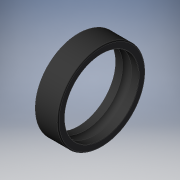
# Autodesk Inventor part: SKF_618/6_PART2
Saved by Autodesk Inventor 2019 (Build 230136000, 136)
## iProperties
Created: 2022-10-05
Part Number: SKF_618/6_PART2
Material: Generic
Catalog Web Link: www.cadenas.de
Description: -Deep groove ball bearings
Vendor: SKF
Document SubType Name: Modeling
Designer: psAdmin
Manufacturer: SKF
Mass: 4 g
Surface Area: 3.38269 cm^2
Volume: 0.123541 cm^3
Density: 1 g/cm^3
Appearance: PSOLRGB-175-175-175
Category: PARTsolutions
Company: SKF
Title: SKF_618/6_PART2
Author: Cadenas PARTsolutions
Comments: Deep groove ball bearings
PSOL_IDENT_0: {$CADENAS_DATA/23d-libs/skf/bearings_units_and_housings/ball_bearings/deep_groove_ball_bearings/bb1_
PSOL_IDENT_1: 001_101.prj},196 {VTYP=3D},{NB=SKF_618/6_PART2},{LINA=SKF_618/6_PART2},{NN=BB1_001_101_PART2},{NOPRJ=
PSOL_IDENT_2: TRUE},{DATE=09.09.2022 10:31:03},{GEOMDATE=07.09.2022 12:28:28},{VERSION=},{LINEID=8510},{WBVAR=},{W
PSOL_IDENT_3: BNUMERIC=}  {NB=SKF_618/6_PART2},{LINA=SKF_618/6_PART2},{KT=DUMMY},{DESIGNATION=618/6},{R12=0.15},{D
PSOL_IDENT_4: D=6.000},{D=13.000},{B=3.500},{C=},{CX=},{CXX=},{CA=0.000},{XXVARIANT=},{XXDESIGN=Single row},{XXSEA
PSOL_IDENT_5: LING=No seals},{DESIGN=dgbb1},{DESIGNIR=dgbb1},{VARIANT=},{DD1=8.00},{DD2=},{DD2X=},{DD2A=0.00},{D1=
PSOL_IDENT_6: 11.00},{D1X=0.00},{D2=},{D2A=0.00},{D3=},{D3X=},{D3A=0.000},{D4=},{HH=0.000},{BB=0.000},{BBX=},{BBA=
PSOL_IDENT_7: 0.000},{FF=},{R0MAX=0.000},{R0=0.000},{PITCH=9.50},{DW=2.000},{DDAMIN=6.800},{DDAMAX=0.000},{DDBMIN=
PSOL_IDENT_8: 0.000},{DDBMAX=0.000},{DBMIN=0.000},{DAMAX=12.200},{BBAMIN=0.000},{CAMAX=0.000},{RAMAX=0.100},{LOAD1=
PSOL_IDENT_9: 0.715},{LOAD2=0.224},{LOAD3=0.010},{SPEED1=110000},{SPEED2=67000},{KR=0.015},{F0=7.000},{Z=8},{II=1}
PSOL_IDENT_10: ,{MASS=0.004},{BEARING=618/6},{RING=},{HELP=1.000},{HELP2=1.000},{DD1ALG=4.000},{YALG=4.000},{PITCH1=
PSOL_IDENT_11: 9.500},{DW1=2.000},{YALG1=5.500},{HALG1=1.000},{SH=4.000},{CU=0.300},{HALG=1},{B1=0},{SHIELDHELP=1},
PSOL_IDENT_12: {D4A=0.000},{FFA=0.000},{RS1=},{HELP3=0},{SUPPRESS=0}
NB: SKF_618/6_PART2
NT: Deep groove ball bearings
NBSYN: SKF_$DESIGNATION._PART2
LINA: SKF_618/6_PART2
CATALOG: SKF
DESIGNATION: 618/6
R12: 0.15
DD: 6
D: 13
B: 3.5
XXDESIGN: Single row
XXSEALING: No seals
LOAD1: 0.715
LOAD2: 0.224
LOAD3: 0.01
SPEED1: 110000
SPEED2: 67000
BEARING: 618/6
SUPPLIER: SKF
ARTICLENO: SKF_618/6_PART2
BOMINFO: SKF_618/6_PART2
CREATOR: CADENAS GmbH
Autodesk Inventor part; units mm, degrees
ref_plane "YZ Plane" through (0, 0, 0) normal (1, 0, 0) x (0, 1, 0)
ref_plane "XZ Plane" through (0, 0, 0) normal (0, 1, 0) x (-1, 0, 0)
ref_plane "XY Plane" through (0, 0, 0) normal (0, 0, 1) x (1, 0, 0)
sketch "Sketch_1" plane through (0, 0, 0) normal (0, 0, 1) x (1, 0, 0)
  line L0 (50, 0) -> (-50, 0)
  line L1 (0, 6.35) -> (0, 5.55)
  arc A0 (0, 5.55) -> (0.05, 5.5) centre (0.05, 5.55) ccw
  line L2 (0.05, 5.5) -> (1.0886, 5.5)
  arc A1 (2.4114, 5.5) -> (1.0886, 5.5) centre (1.75, 4.75) ccw
  line L3 (2.4114, 5.5) -> (3.45, 5.5)
  arc A2 (3.45, 5.5) -> (3.5, 5.55) centre (3.45, 5.55) ccw
  line L4 (3.5, 5.55) -> (3.5, 6.35)
  arc A3 (3.5, 6.35) -> (3.35, 6.5) centre (3.35, 6.35) ccw
  line L5 (3.35, 6.5) -> (0.15, 6.5)
  arc A4 (0.15, 6.5) -> (0, 6.35) centre (0.15, 6.35) ccw
  constraints: 12 end point, 10 point on circle, 5 centre point
revolve "Revolution1" add sketch "Sketch_1" angle 360 about axis through (50, 0, 0) along (1, 0, 0)
body "Solid1"
